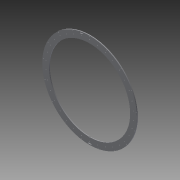
# Autodesk Inventor part: laser circle 3D
Saved by Autodesk Inventor 2013 (Build 170138000, 138)
## iProperties
Created: 2013-07-18
Part Number: laser circle 3D
Material: Generic
Document SubType Name: Modeling
Designer: owner
Density: 1 g/cm^3
Author: owner
Autodesk Inventor part; units mm, degrees
ref_plane "YZ Plane" through (0, 0, 0) normal (1, 0, 0) x (0, 1, 0)
ref_plane "XZ Plane" through (0, 0, 0) normal (0, 1, 0) x (-1, 0, 0)
ref_plane "XY Plane" through (0, 0, 0) normal (0, 0, 1) x (1, 0, 0)
sketch "Sketch1" plane through (0, 0, 0) normal (0, 0, 1) x (1, 0, 0)
  circle A0 centre (0, 0) radius 355.6
  circle A1 centre (0, 0) radius 304.8
  circle A2 centre (0, 330.2) radius 3.175
  circle A3 centre (0, 349.25) radius 3.175
  circle A4 centre (119.282, 307.9023) radius 3.175
  circle A5 centre (126.1637, 325.6659) radius 3.175
  circle A6 centre (222.4543, 244.0207) radius 3.175
  circle A7 centre (235.2882, 258.0989) radius 3.175
  circle A8 centre (295.5829, 147.1828) radius 3.175
  circle A9 centre (312.6358, 155.6741) radius 3.175
  circle A10 centre (328.7914, 30.467) radius 3.175
  circle A11 centre (347.7602, 32.2247) radius 3.175
  circle A12 centre (317.5948, -90.3635) radius 3.175
  circle A13 centre (335.9176, -95.5768) radius 3.175
  circle A14 centre (263.5053, -198.99) radius 3.175
  circle A15 centre (278.7075, -210.4701) radius 3.175
  circle A16 centre (173.8279, -280.7417) radius 3.175
  circle A17 centre (183.8564, -296.9383) radius 3.175
  circle A18 centre (60.6741, -324.5777) radius 3.175
  circle A19 centre (64.1745, -343.3034) radius 3.175
  circle A20 centre (-60.6741, -324.5777) radius 3.175
  circle A21 centre (-64.1745, -343.3034) radius 3.175
  circle A22 centre (-173.8279, -280.7417) radius 3.175
  circle A23 centre (-183.8564, -296.9383) radius 3.175
  circle A24 centre (-263.5053, -198.99) radius 3.175
  circle A25 centre (-278.7075, -210.4701) radius 3.175
  circle A26 centre (-317.5948, -90.3635) radius 3.175
  circle A27 centre (-335.9176, -95.5768) radius 3.175
  circle A28 centre (-328.7914, 30.467) radius 3.175
  circle A29 centre (-347.7602, 32.2247) radius 3.175
  circle A30 centre (-295.5829, 147.1828) radius 3.175
  circle A31 centre (-312.6358, 155.6741) radius 3.175
  circle A32 centre (-222.4543, 244.0207) radius 3.175
  circle A33 centre (-235.2882, 258.0989) radius 3.175
  circle A34 centre (-119.282, 307.9023) radius 3.175
  circle A35 centre (-126.1637, 325.6659) radius 3.175
  circle A36 centre (0, -330.2) radius 3.175
  line L0 (0, -308.356) -> (3.302, -308.356)
  line L1 (0, -308.356) -> (-3.175, -308.356)
  line L2 (3.302, -308.356) -> (3.302, -304.7821)
  line L3 (-3.175, -308.356) -> (-3.175, -304.7835)
  circle A37 centre (119.282, -307.9023) radius 3.175
  line L4 (111.391, -287.5334) -> (114.4701, -286.3406)
  line L5 (111.391, -287.5334) -> (108.4304, -288.6803)
  line L6 (114.4701, -286.3406) -> (113.179, -283.008)
  line L7 (108.4304, -288.6803) -> (107.1399, -285.3491)
  circle A38 centre (222.4543, -244.0207) radius 3.175
  line L8 (207.7381, -227.8778) -> (210.1783, -225.6533)
  line L9 (207.7381, -227.8778) -> (205.3917, -230.0168)
  line L10 (210.1783, -225.6533) -> (207.7706, -223.0122)
  line L11 (205.3917, -230.0168) -> (202.9849, -227.3767)
  circle A39 centre (295.5829, -147.1828) radius 3.175
  line L12 (276.029, -137.4461) -> (277.5008, -134.4903)
  line L13 (276.029, -137.4461) -> (274.6138, -140.2882)
  line L14 (277.5008, -134.4903) -> (274.3016, -132.8972)
  line L15 (274.6138, -140.2882) -> (271.4157, -138.6958)
  circle A40 centre (328.7914, -30.467) radius 3.175
  line L16 (307.0406, -28.4515) -> (307.3453, -25.1636)
  line L17 (307.0406, -28.4515) -> (306.7477, -31.613)
  line L18 (307.3453, -25.1636) -> (303.7866, -24.8338)
  line L19 (306.7477, -31.613) -> (303.1904, -31.2833)
  circle A41 centre (317.5948, 90.3635) radius 3.175
  line L20 (296.5847, 84.3856) -> (295.6811, 87.5616)
  line L21 (296.5847, 84.3856) -> (297.4536, 81.3318)
  line L22 (295.6811, 87.5616) -> (292.2436, 86.5835)
  line L23 (297.4536, 81.3318) -> (294.0174, 80.3542)
  circle A42 centre (263.5053, 198.99) radius 3.175
  line L24 (246.0734, 185.826) -> (244.0835, 188.4611)
  line L25 (246.0734, 185.826) -> (247.9868, 183.2923)
  line L26 (244.0835, 188.4611) -> (241.2315, 186.3073)
  line L27 (247.9868, 183.2923) -> (245.1358, 181.1394)
  circle A43 centre (173.8279, 280.7417) radius 3.175
  line L28 (162.3285, 262.1696) -> (159.5211, 263.9078)
  line L29 (162.3285, 262.1696) -> (165.028, 260.4981)
  line L30 (159.5211, 263.9078) -> (157.6397, 260.8693)
  line L31 (165.028, 260.4981) -> (163.1473, 257.4607)
  circle A44 centre (60.6741, 324.5777) radius 3.175
  line L32 (56.6603, 303.1057) -> (53.4145, 303.7124)
  line L33 (56.6603, 303.1057) -> (59.7812, 302.5222)
  line L34 (53.4145, 303.7124) -> (52.7578, 300.1994)
  line L35 (59.7812, 302.5222) -> (59.1248, 299.0105)
  circle A45 centre (-60.6741, 324.5777) radius 3.175
  line L36 (-56.6603, 303.1057) -> (-59.906, 302.4989)
  line L37 (-56.6603, 303.1057) -> (-53.5393, 303.6891)
  line L38 (-59.906, 302.4989) -> (-59.2493, 298.9859)
  line L39 (-53.5393, 303.6891) -> (-52.8829, 300.1774)
  circle A46 centre (-173.8279, 280.7417) radius 3.175
  line L40 (-162.3285, 262.1696) -> (-165.1359, 260.4313)
  line L41 (-162.3285, 262.1696) -> (-159.6291, 263.841)
  line L42 (-165.1359, 260.4313) -> (-163.2545, 257.3927)
  line L43 (-159.6291, 263.841) -> (-157.7484, 260.8035)
  circle A47 centre (-263.5053, 198.99) radius 3.175
  line L44 (-246.0734, 185.826) -> (-248.0633, 183.191)
  line L45 (-246.0734, 185.826) -> (-244.16, 188.3597)
  line L46 (-248.0633, 183.191) -> (-245.2113, 181.0372)
  line L47 (-244.16, 188.3597) -> (-241.3091, 186.2068)
  circle A48 centre (-317.5948, 90.3635) radius 3.175
  line L48 (-296.5847, 84.3856) -> (-297.4883, 81.2097)
  line L49 (-296.5847, 84.3856) -> (-295.7158, 87.4394)
  line L50 (-297.4883, 81.2097) -> (-294.0509, 80.2316)
  line L51 (-295.7158, 87.4394) -> (-292.2797, 86.4618)
  circle A49 centre (-328.7914, -30.467) radius 3.175
  line L52 (-307.0406, -28.4515) -> (-306.7359, -31.7394)
  line L53 (-307.0406, -28.4515) -> (-307.3336, -25.29)
  line L54 (-306.7359, -31.7394) -> (-303.1773, -31.4097)
  line L55 (-307.3336, -25.29) -> (-303.7763, -24.9604)
  circle A50 centre (-295.5829, -147.1828) radius 3.175
  line L56 (-276.029, -137.4461) -> (-274.5571, -140.4019)
  line L57 (-276.029, -137.4461) -> (-277.4442, -134.604)
  line L58 (-274.5571, -140.4019) -> (-271.3579, -138.8089)
  line L59 (-277.4442, -134.604) -> (-274.2462, -133.0115)
  circle A51 centre (-222.4543, -244.0207) radius 3.175
  line L60 (-207.7381, -227.8778) -> (-205.2979, -230.1024)
  line L61 (-207.7381, -227.8778) -> (-210.0844, -225.7389)
  line L62 (-205.2979, -230.1024) -> (-202.8902, -227.4612)
  line L63 (-210.0844, -225.7389) -> (-207.6776, -223.0987)
  circle A52 centre (-119.282, -307.9023) radius 3.175
  line L64 (-111.391, -287.5334) -> (-108.312, -288.7262)
  line L65 (-111.391, -287.5334) -> (-114.3516, -286.3865)
  line L66 (-108.312, -288.7262) -> (-107.021, -285.3937)
  line L67 (-114.3516, -286.3865) -> (-113.0611, -283.0552)
  line L68 (0, -342.9) -> (12.7, -342.9)
  line L69 (12.7, -342.9) -> (12.7, -349.25)
  line L70 (12.7, -349.25) -> (-12.7, -349.25)
  line L71 (-12.7, -349.25) -> (-12.7, -342.9)
  line L72 (-12.7, -342.9) -> (0, -342.9)
  line L73 (-63.0181, 337.0595) -> (-75.5018, 334.7255)
  line L74 (-75.5018, 334.7255) -> (-76.6688, 340.9674)
  line L75 (-76.6688, 340.9674) -> (-51.7014, 345.6354)
  line L76 (-51.7014, 345.6354) -> (-50.5344, 339.3935)
  line L77 (-50.5344, 339.3935) -> (-63.0181, 337.0595)
  circle A53 centre (0, 0) radius 304.8
  dimension "d1" = 711.2
  dimension "d3" = 609.6
  dimension "d6" = 6.35
  dimension "d7" = 6.35
  dimension "d10" = 360
  dimension "d13" = 6.35
  dimension "d15" = 3.302
  dimension "d18" = 360
  dimension "d20" = 342.9
  dimension "d21" = 12.7
  dimension "d22" = 6.35
  dimension "d23" = 25.4
  dimension "d26" = 360
  constraints: 156 end point, 53 centre point, 3 coincident, 2 parallel, 2 point on circle, 1 collinear, 1 perpendicular, 261 other
  measures "d1" diameter of A0
  measures "d3" diameter of A1
  measures "d6" diameter of A2
  measures "d7" diameter of A3
  measures "d13" diameter of A36
  measures "d15" distance of L0.start L0.end
  measures "d20" distance of A1.centre L68.start
  measures "d21" distance of L68.start L68.end
  measures "d22" distance of L68.end L69.end
  measures "d23" distance of L69.end L70.end
extrude "Extrusion1" add sketch "Sketch1" along normal blind 6.35 contours A0 | A1 L22 L20 L21 L23 | L18 L16 L17 L19 A1 | A1 L26 L24 L25 L27 | L14 L12 L13 L15 A1 | A1 L30 L28 L29 L31 | L10 L8 L9 L11 A1 | A1 L34 L32 L33 L35 | L6 L4 L5 L7 A1 | A1 L38 L36 L37 L39 | A1 L42 L40 L41 L43 | L66 L64 L65 L67 A1 | A1 L46 L44 L45 L47 | L62 L60 L61 L63 A1 | A1 L50 L48 L49 L51 | L58 L56 L57 L59 A1 | A1 L54 L52 L53 L55
body "Solid1"
